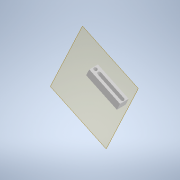
# Autodesk Inventor part: s_support
Saved by Autodesk Inventor 2020.1 (Build 241239000, 239)
## iProperties
Created: 2019-10-17
Part Number: s_support
Material: Generic
Document SubType Name: Modeling
Designer: jesse
Density: 1 g/cm^3
Appearance: Default
support_length: 2.300 in
hole_size: 0.118 in
Author: jesse
Autodesk Inventor part; units mm, degrees
ref_plane "YZ Plane" through (0, 0, 0) normal (1, 0, 0) x (0, 1, 0)
ref_plane "XZ Plane" through (0, 0, 0) normal (0, 1, 0) x (-1, 0, 0)
ref_plane "XY Plane" through (0, 0, 0) normal (0, 0, 1) x (1, 0, 0)
ref_plane "Work Plane1" through (19.722, 36.341, 0) normal (0, 0, 1) x (0.4250843, 0.9051538, 0)
sketch "Sketch1" plane through (19.722, 36.341, 0) normal (0, 0, 1) x (0.4250843, 0.9051538, 0)
  line L0 (-12.1227, 70.1452) -> (-18.8796, 70.1452)
  line L1 (-18.8796, 70.1452) -> (-18.8796, 11.7252)
  line L2 (-18.8796, 11.7252) -> (-12.1227, 11.7252)
  line L3 (-12.1227, 11.7252) -> (-12.1227, 70.1452)
  point P0 (-41.2777, 2.4034)
  dimension "support_length" = 58.42
  constraints: 8 end point, 2 parallel, 1 horizontal, 1 perpendicular
  measures "support_length" distance of L2.end L0.start
extrude "Extrusion1" add sketch "Sketch1" along normal blind 8
sketch "Sketch2" plane through (1.0834, 24.2363, 0) normal (-0.4250843, -0.9051538, 0) x (0, 0, 1)
  line L0 (0, 58.42) -> (8, 58.42) construction
  line L1 (4, 58.42) -> (4, 0) construction
  line L2 (0, 0) -> (8, 0) construction
  line L3 (4, 52.42) -> (4, 2) construction
  line L4 (2.5, 52.42) -> (2.5, 2)
  line L5 (5.5, 2) -> (5.5, 52.42)
  arc A0 (5.5, 52.42) -> (2.5, 52.42) centre (4, 52.42) ccw
  arc A1 (2.5, 2) -> (5.5, 2) centre (4, 2) ccw
  line L6 (4, 2) -> (6.3728, 2) construction
  line L7 (4, 52.42) -> (6.6371, 52.42) construction
  line L8 (5.634, 2) -> (5.634, 0) construction
  circle A2 centre (4, 56.42) radius 1.5
  line L9 (4, 56.42) -> (7.1435, 56.42) construction
  point P0 (0, -9.3218)
  point P1 (4, 27.21)
  dimension "d5" = 3
  dimension "d6" = 3
  dimension "d7" = 2
  dimension "d8" = 2
  dimension "d9" = 4
  constraints: 18 end point, 5 point on line, 4 point on circle, 4 tangent, 3 centre point, 3 horizontal, 3 midpoint, 1 parallel
  measures "d5" distance between parallel lines of L4 L5
  measures "d6" diameter of A2
  measures "d7" distance between parallel lines of L9 L0
  measures "d8" distance between parallel lines of L6 L2
  measures "d9" distance between parallel lines of L7 L9
extrude "Extrusion2" cut sketch "Sketch2" against normal blind 15.875
equation "\"d5\" = hole_size"
equation "\"d6\" = hole_size"
equation "\"hole_size\" = 3"
body "Solid1"
